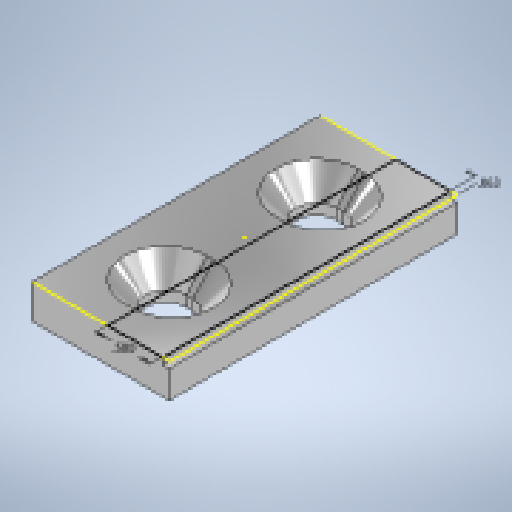
# Autodesk Inventor part: Jaw
Saved by Autodesk Inventor 2023.2 (Build 272271000, 271)
## iProperties
Created: 2024-03-01
Part Number: Jaw
Material: Aluminum 6061
Document SubType Name: Modeling
Designer: Nathan Cai
Density: 2.7 g/cm^3
Appearance: Aluminum - Flat
Author: Nathan Cai
Autodesk Inventor part; units mm, degrees
ref_plane "YZ Plane" through (0, 0, 0) normal (1, 0, 0) x (0, 1, 0)
ref_plane "XZ Plane" through (0, 0, 0) normal (0, 1, 0) x (-1, 0, 0)
ref_plane "XY Plane" through (0, 0, 0) normal (0, 0, 1) x (1, 0, 0)
sketch "Sketch1" plane through (0, 0, 0) normal (0, 1, 0) x (-1, 0, 0)
  line L0 (-25.4, 31.75) -> (25.4, 31.75)
  line L1 (25.4, 31.75) -> (25.4, -31.75)
  line L2 (25.4, -31.75) -> (-25.4, -31.75)
  line L3 (-25.4, -31.75) -> (-25.4, 31.75)
  line L4 (-25.4, 31.75) -> (25.4, -31.75) construction
  line L5 (25.4, 31.75) -> (-25.4, -31.75) construction
  line L6 (0, 31.75) -> (0, -31.75) construction
  line L7 (-0.7937, -17.4625) -> (0.7938, -17.4625) construction
  line L8 (-0.7937, -23.0187) -> (0.7938, -23.0187)
  line L9 (0.7938, -11.9063) -> (-0.7937, -11.9063)
  arc A0 (-0.7937, -11.9063) -> (-0.7937, -23.0187) centre (-0.7937, -17.4625) ccw
  arc A1 (0.7938, -23.0187) -> (0.7938, -11.9063) centre (0.7938, -17.4625) ccw
  line L10 (25.4, 0) -> (-25.4, 0) construction
  line L11 (-0.7937, 17.4625) -> (0.7937, 17.4625) construction
  line L12 (-0.7938, 23.0187) -> (0.7937, 23.0187)
  line L13 (0.7938, 11.9063) -> (-0.7937, 11.9063)
  arc A2 (-0.7938, 23.0187) -> (-0.7937, 11.9063) centre (-0.7937, 17.4625) ccw
  arc A3 (0.7938, 11.9063) -> (0.7937, 23.0187) centre (0.7937, 17.4625) ccw
  circle A4 centre (0, 17.4625) radius 5.5562
  circle A5 centre (0, -17.4625) radius 5.5562
  point P0 (0, 0)
  point P1 (0, 0)
  point P2 (0, -11.9063)
  point P3 (0, -23.0187)
  point P4 (0, 11.9063)
  point P5 (0, 23.0187)
  dimension "d0" = 50.8
  dimension "d1" = 63.5
  dimension "d2" = 0.7937
  dimension "d3" = 11.1125
  dimension "d4" = 17.4625
  constraints: 32 end point, 8 midpoint, 8 point on circle, 7 symmetric about line, 6 centre point, 6 tangent, 3 parallel, 2 coincident, 2 perpendicular, 1 horizontal, 1 point on line, 2 other
  measures "d0" distance of L1.end L2.end
  measures "d1" distance of L0.end L1.end
  measures "d2" distance of point (0, -17.463) L7.end
  measures "d3" diameter of A1
  measures "d4" distance from line of point (0, 0) L7
extrude "Extrusion1" add sketch "Sketch1" along normal blind 11.1125 contours L0 L1 L2 L3 | A0 L9 A5 L8 | A5 L9 A1 L8 | L12 A4 L13 A2 | L12 A3 L13 A4
sketch "Sketch2" plane through (0, 11.1125, 0) normal (0, 1, 0) x (1, 0, 0)
  line L0 (25.4, 31.75) -> (-25.4, 31.75) projected
  line L1 (-25.4, -31.75) -> (25.4, -31.75) projected
  line L2 (23.8125, 31.75) -> (11.1125, 31.75)
  line L3 (11.1125, 31.75) -> (11.1125, -31.75)
  line L4 (11.1125, -31.75) -> (23.8125, -31.75)
  line L5 (23.8125, -31.75) -> (23.8125, 31.75)
  line L6 (25.4, -31.75) -> (25.4, 31.75) projected
  point P0 (0, 0)
  point P1 (23.8125, -31.75)
  dimension "d7" = 12.7
  dimension "d8" = 1.5875
  constraints: 8 end point, 2 parallel, 2 point on line, 1 horizontal, 1 perpendicular
  measures "d7" distance of L4.end L3.end
  measures "d8" distance between parallel lines of L6 L5
extrude "Extrusion3" cut sketch "Sketch2" against normal blind 1.5875 contours L6 L1 L5 L0
chamfer "Chamfer1" distance 4.7625 angle 49 2 edges at (0, 11.1125, 23.0188) (0, 11.1125, -23.0188) measured on face at (-18.6651, 11.1125, -5.1641)
extrude "Extrusion4" cut sketch "Sketch2" against normal blind 4.7625 contours L5 L1 L3 L0
extrude "Extrusion5" cut sketch "Sketch1" along normal blind 7.9375 contours A0 L9 A5 L8 | A5 L9 A1 L8 | A5 | L12 A4 L13 A2 | L12 A3 L13 A4 | A4
body "Solid1"
